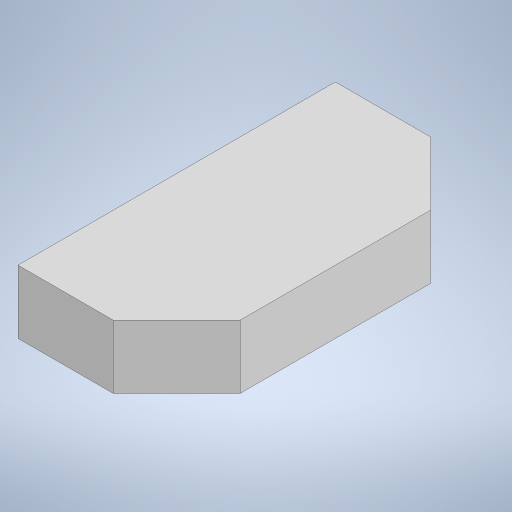
# Autodesk Inventor part: 책상 고정 판
Saved by Autodesk Inventor 2023 (Build 270158000, 158)
## iProperties
Created: 2022-11-11
Part Number: 책상 고정 판
Material: 일반
Document SubType Name: Modeling
Designer: hyunsu
Density: 1 g/cm^3
Appearance: 기본값
Author: hyunsu
Autodesk Inventor part; units mm, degrees
ref_plane "YZ Plane" through (0, 0, 0) normal (1, 0, 0) x (0, 1, 0)
ref_plane "XZ Plane" through (0, 0, 0) normal (0, 1, 0) x (-1, 0, 0)
ref_plane "XY Plane" through (0, 0, 0) normal (0, 0, 1) x (1, 0, 0)
sketch "스케치1" plane through (0, 0, 0) normal (0, 1, 0) x (-1, 0, 0)
  line L0 (12.5, 25) -> (-12.5, 25)
  line L1 (-12.5, 25) -> (-12.5, -25)
  line L2 (-12.5, -25) -> (12.5, -25)
  line L3 (12.5, -25) -> (12.5, 25)
  line L4 (12.5, 25) -> (-12.5, -25) construction
  line L5 (-12.5, 25) -> (12.5, -25) construction
  point P0 (0, 0)
  dimension "d0" = 50
  dimension "d1" = 25
  constraints: 12 end point, 2 midpoint, 2 parallel, 1 horizontal, 1 perpendicular
  measures "d0" distance of L2.end L0.start
  measures "d1" distance of L1.end L2.end
extrude "돌출1" add sketch "스케치1" along normal blind 10
chamfer "모따기1" distance 10 angle 45 2 edges at (12.5, 5, -25) (12.5, 5, 25)
sketch "스케치2" plane through (0, 0, 0) normal (0, -1, 0) x (1, 0, 0)
  circle A0 centre (0.5, 0) radius 8
  line L0 (12.5, 15) -> (12.5, -15) projected
  point P0 (0, 0)
  point P1 (12.5, 0)
  point P2 (12.5, 0)
  dimension "d7" = 16
  dimension "d8" = 12
  constraints: 2 horizontal alignment, 2 midpoint, 1 centre point
  measures "d7" diameter of A0
  measures "d8" distance from line of L0 A0.centre
extrude "돌출2" cut sketch "스케치2" against normal blind 7
sketch "스케치3" plane through (0, 0, 0) normal (0, -1, 0) x (1, 0, 0)
  circle A0 centre (0, 10.5) radius 1
  line L0 (0, 0) -> (5.1796, 0)
  circle A1 centre (-10.5, 0) radius 1
  circle A2 centre (0, -10.5) radius 1
  circle A3 centre (10.5, 0) radius 1
  dimension "d11" = 2
  dimension "d18" = 360
  dimension "d20" = 21
  constraints: 4 centre point, 2 end point, 1 horizontal, 9 other
  measures "d11" diameter of A0
  measures "d20" distance of A2.centre A0.centre
extrude "돌출3" cut sketch "스케치3" against normal blind 7
